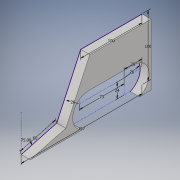
# Autodesk Inventor part: Side Plate
Saved by Autodesk Inventor 2019 (Build 230136000, 136)
## iProperties
Created: 2019-09-06
Part Number: Side Plate
Material: Generic
Document SubType Name: Modeling
Designer: isaac
Density: 1 g/cm^3
Appearance: Default
Author: isaac
Autodesk Inventor part; units mm, degrees
ref_plane "YZ Plane" through (0, 0, 0) normal (1, 0, 0) x (0, 1, 0)
ref_plane "XZ Plane" through (0, 0, 0) normal (0, 1, 0) x (-1, 0, 0)
ref_plane "XY Plane" through (0, 0, 0) normal (0, 0, 1) x (1, 0, 0)
sketch "Sketch2" plane through (0, 0, 0) normal (1, 0, 0) x (0, 1, 0)
  line L0 (0, 0) -> (100, 0)
  line L1 (100, 0) -> (100, 100)
  line L2 (0, 0) -> (0, 197) construction
  line L3 (0, 197) -> (15.5291, 139.0445)
  line L4 (0, 197) -> (60, 197) construction
  line L5 (15.5291, 139.0445) -> (100, 100)
  line L6 (0, 0) -> (24, 0) construction
  line L7 (24, 0) -> (24, 29) construction
  line L8 (24, 29) -> (0, 29) construction
  line L9 (0, 29) -> (0, 0) construction
  line L10 (24, 29) -> (24, 102) construction
  arc A0 (0, 19) -> (50, 29) centre (24, 29) ccw
  line L11 (0, 0) -> (0, 19)
  arc A1 (50, 102) -> (0, 112) centre (24, 102) ccw
  line L12 (24, 102) -> (50, 102) construction
  line L13 (24, 29) -> (50, 29) construction
  line L14 (50, 29) -> (50, 102)
  line L15 (0, 112) -> (0, 197)
  dimension "d10" = 100
  dimension "d11" = 100
  dimension "d12" = 197
  dimension "d13" = 60
  dimension "d14" = 75
  dimension "d15" = 24
  dimension "d16" = 29
  dimension "d17" = 73
  dimension "d18" = 26
  dimension "d19" = 26
  constraints: 32 end point, 4 horizontal, 4 point on circle, 3 parallel, 3 vertical, 2 centre point, 2 coincident, 2 point on line, 1 collinear, 1 equal length, 1 perpendicular
  measures "d10" distance of L0.start L0.end
  measures "d11" distance of L0.end L1.end
  measures "d12" distance of L0.start L2.end
  measures "d13" distance of L2.end L3.end
  measures "d14" angle of L3 L4
  measures "d15" distance of L8.end L7.end
  measures "d16" distance of L7.end L6.end
  measures "d17" distance of L7.end L10.end
  measures "d18" radius of A0
  measures "d19" radius of A1
extrude "Extrusion1" add sketch "Sketch2" along normal blind 15
body "Solid1"
